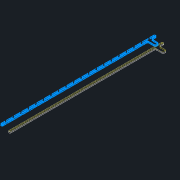
# Autodesk Inventor part: belt1
Saved by Autodesk Inventor 2022 (Build 260153000, 153)
## iProperties
Created: 2022-05-04
Part Number: belt1
Material: ゴム
Document SubType Name: Modeling
Designer: Yuta Kage
Density: 0.93 g/cm^3
Appearance: ゴム - 黒
Mass: 38.4563 g
Surface Area: 1281.35 cm^2
Volume: 41.3509 cm^3
Author: Yuta Kage
Autodesk Inventor part; units mm, degrees
ref_plane "YZ Plane" through (0, 0, 0) normal (1, 0, 0) x (0, 1, 0)
ref_plane "XZ Plane" through (0, 0, 0) normal (0, 1, 0) x (-1, 0, 0)
ref_plane "XY Plane" through (0, 0, 0) normal (0, 0, 1) x (1, 0, 0)
sketch "スケッチ1" plane through (0, 0, 0) normal (0, 1, 0) x (-1, 0, 0)
  arc A0 (-9.5493, 0) -> (9.5493, 0) centre (0, 0) ccw construction
  arc A1 (9.5493, 1400) -> (-9.5493, 1400) centre (0, 1400) ccw construction
  arc A2 (-63.925, 72.1887) -> (-63.925, 37.8113) centre (-63.925, 55) ccw construction
  arc A3 (-9.5493, 28.4353) -> (-18.9253, 37.8113) centre (-18.9253, 28.4353) ccw construction
  arc A4 (-18.9253, 72.1887) -> (-9.5493, 81.5647) centre (-18.9253, 81.5647) ccw construction
  line L0 (-63.925, 37.8113) -> (-18.9253, 37.8113) construction
  line L1 (-9.5493, 28.4353) -> (-9.5493, 0) construction
  line L2 (9.5493, 0) -> (9.5493, 1400) construction
  line L3 (-9.5493, 1400) -> (-9.5493, 81.5647) construction
  line L4 (-18.9253, 72.1887) -> (-63.925, 72.1887) construction
  line L5 (9.9253, 1400) -> (9.9253, 0)
  arc A5 (-9.9253, 0) -> (9.9253, 0) centre (0, 0) ccw
  line L6 (-9.9253, 0) -> (-9.9253, 28.4353)
  arc A6 (-9.9253, 28.4353) -> (-18.9253, 37.4353) centre (-18.9253, 28.4353) ccw
  line L7 (-18.9253, 37.4353) -> (-63.925, 37.4353)
  arc A7 (-63.925, 72.5647) -> (-63.925, 37.4353) centre (-63.925, 55) ccw
  line L8 (-63.925, 72.5647) -> (-18.9253, 72.5647)
  arc A8 (-18.9253, 72.5647) -> (-9.9253, 81.5647) centre (-18.9253, 81.5647) ccw
  line L9 (-9.9253, 81.5647) -> (-9.9253, 1400)
  arc A9 (9.9253, 1400) -> (-9.9253, 1400) centre (0, 1400) ccw
  line L10 (9.2953, 1400) -> (9.2953, 0)
  arc A10 (-9.2953, 0) -> (9.2953, 0) centre (0, 0) ccw
  line L11 (-9.2953, 0) -> (-9.2953, 28.4353)
  arc A11 (-9.2953, 28.4353) -> (-18.9253, 38.0653) centre (-18.9253, 28.4353) ccw
  line L12 (-18.9253, 38.0653) -> (-63.925, 38.0653)
  arc A12 (-63.925, 71.9347) -> (-63.925, 38.0653) centre (-63.925, 55) ccw
  line L13 (-63.925, 71.9347) -> (-18.9253, 71.9347)
  arc A13 (-18.9253, 71.9347) -> (-9.2953, 81.5647) centre (-18.9253, 81.5647) ccw
  line L14 (-9.2953, 81.5647) -> (-9.2953, 1400)
  arc A14 (9.2953, 1400) -> (-9.2953, 1400) centre (0, 1400) ccw
  circle A15 centre (-18.9253, 81.5647) radius 9 construction
  circle A16 centre (-18.9253, 28.4353) radius 9 construction
  dimension "d10" = 18
  dimension "d0" = 19.0986
  dimension "d1" = 19.0986
  dimension "d2" = 34.3775
  dimension "d3" = 1400
  dimension "d4" = 55
  dimension "d5" = 63.925
  dimension "d6" = 0.254
  dimension "d7" = 0.63
  dimension "d14" = 28.4353
  constraints: 30 end point, 30 point on circle, 15 centre point, 9 tangent, 6 parallel, 6 perpendicular, 3 coincident, 3 horizontal alignment, 2 vertical alignment, 22 other
  measures "d0" diameter of A0
  measures "d1" diameter of A1
  measures "d2" diameter of A2
  measures "d3" distance of A1.centre point (0, 0)
  measures "d4" vertical distance of point (0, 0) A2.centre
  measures "d5" horizontal distance of point (0, 0) A2.centre
  measures "d6" distance between parallel lines of L2 L10
  measures "d7" distance between parallel lines of L10 L5
  measures "d14" vertical distance of point (0, 0) A3.centre
extrude "押し出し1" add sketch "スケッチ1" along normal mid plane 10
sketch "スケッチ2" plane through (0, 5, 0) normal (0, 1, 0) x (1, 0, 0)
  line L0 (63.925, -37.4353) -> (18.9253, -37.4353) projected
  arc A0 (9.9253, -28.4353) -> (18.9253, -37.4353) centre (18.9253, -28.4353) ccw projected
  line L1 (9.9253, -28.4353) -> (9.9253, 0) projected
  arc A1 (9.9253, 0) -> (-9.9253, 0) centre (0, 0) ccw projected
  line L2 (-9.9253, 0) -> (-9.9253, -1400) projected
  arc A2 (-9.9253, -1400) -> (9.9253, -1400) centre (0, -1400) ccw projected
  line L3 (9.9253, -1400) -> (9.9253, -81.5647) projected
  arc A3 (18.9253, -72.5647) -> (9.9253, -81.5647) centre (18.9253, -81.5647) ccw projected
  line L4 (18.9253, -72.5647) -> (63.925, -72.5647) projected
  arc A4 (63.925, -72.5647) -> (63.925, -37.4353) centre (63.925, -55) ccw projected
  line L5 (63.925, -71.9347) -> (18.9253, -71.9347) projected
  arc A5 (18.9253, -71.9347) -> (9.2953, -81.5647) centre (18.9253, -81.5647) ccw projected
  line L6 (9.2953, -81.5647) -> (9.2953, -1400) projected
  arc A6 (-9.2953, -1400) -> (9.2953, -1400) centre (0, -1400) ccw projected
  line L7 (-9.2953, -1400) -> (-9.2953, 0) projected
  arc A7 (9.2953, 0) -> (-9.2953, 0) centre (0, 0) ccw projected
  line L8 (9.2953, 0) -> (9.2953, -28.4353) projected
  arc A8 (9.2953, -28.4353) -> (18.9253, -38.0653) centre (18.9253, -28.4353) ccw projected
  line L9 (18.9253, -38.0653) -> (63.925, -38.0653) projected
  arc A9 (63.925, -71.9347) -> (63.925, -38.0653) centre (63.925, -55) ccw projected
  line L10 (-8.5453, 0) -> (-8.5453, -1400)
  arc A10 (-8.5453, -1400) -> (8.5453, -1400) centre (0, -1400) ccw
  line L11 (8.5453, -1400) -> (8.5453, -81.5647)
  arc A11 (18.9253, -71.1847) -> (8.5453, -81.5647) centre (18.9253, -81.5647) ccw
  line L12 (18.9253, -71.1847) -> (63.925, -71.1847)
  arc A12 (63.925, -71.1847) -> (63.925, -38.8153) centre (63.925, -55) ccw
  line L13 (63.925, -38.8153) -> (18.9253, -38.8153)
  arc A13 (8.5453, -28.4353) -> (18.9253, -38.8153) centre (18.9253, -28.4353) ccw
  line L14 (8.5453, -28.4353) -> (8.5453, 0)
  arc A14 (8.5453, 0) -> (-8.5453, 0) centre (0, 0) ccw
  dimension "d11" = 0.75
  constraints: 10 end point, 10 point on circle, 5 centre point, 9 other
  measures "d11" radial gap between concentric circles of A7 A14
extrude "押し出し2" add sketch "スケッチ2" against normal blind 10 separate body contours L5 A5 L6 A6 L7 A7 L8 A8 L9 A9
equation "\"d1\" = d0"
